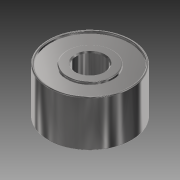
# Autodesk Inventor part: bearing_693
Saved by Autodesk Inventor 2013 (Build 170138000, 138)
## iProperties
Shininess: 86.0
Created: 2011-05-14
Part Number: bearing_693
Document SubType Name: Modeling
Designer: Noa Izumi
Material: Default
Density: 1 g/cm^3
Density: 0.0
Volumn: 0.0
Area: 0.0
PropertySet Name: Model Information
Control State: 0
Master: False
Checked Out: False
Author: Noa Izumi
Autodesk Inventor part; units mm, degrees
ref_plane "YZ Plane" through (0, 0, 0) normal (1, 0, 0) x (0, 1, 0)
ref_plane "XZ Plane" through (0, 0, 0) normal (0, 1, 0) x (-1, 0, 0)
ref_plane "XY Plane" through (0, 0, 0) normal (0, 0, 1) x (1, 0, 0)
sketch "Sketch1" plane through (0, 0, 0) normal (0, 0, 1) x (1, 0, 0)
  circle A0 centre (0, 0) radius 4.5
  circle A1 centre (0, 0) radius 1.5
  dimension "d0" = 9
  dimension "d1" = 3
  constraints: 2 centre point, 1 coincident
  measures "d0" diameter of A0
  measures "d1" diameter of A1
extrude "Extrusion1" add sketch "Sketch1" along normal blind 5
sketch "Sketch2" plane through (0, 0, 5) normal (0, 0, 1) x (1, 0, 0)
  circle A0 centre (0, 0) radius 4.5 projected
  circle A1 centre (0, 0) radius 2.5
  circle A2 centre (0, 0) radius 4.25
  dimension "d4" = 8.5
  dimension "d5" = 5
  constraints: 2 centre point, 2 coincident
  measures "d4" diameter of A2
  measures "d5" diameter of A1
extrude "Extrusion2" cut sketch "Sketch2" against normal blind 0.25 contours A2
sketch "Sketch3" plane through (0, 0, 0) normal (0, 0, -1) x (-1, 0, 0)
  circle A0 centre (0, 0) radius 4.5 projected
  circle A1 centre (0, 0) radius 2.5
  circle A2 centre (0, 0) radius 4.25
  dimension "d8" = 5
  dimension "d9" = 8.5
  constraints: 2 centre point, 2 coincident
  measures "d8" diameter of A1
  measures "d9" diameter of A2
extrude "Extrusion3" cut sketch "Sketch3" against normal blind 0.25 contours A2
fillet "Fillet1" radius 0.125 6 edges at (-4.5, 0, 0) (4.25, 0, 0) (-4.5, 0, 5) (-4.25, 0, 5) (2.5, 0, 0) (-2.5, 0, 5)
chamfer "Chamfer1" distance 0.125 angle 45 2 edges at (-1.5, 0, 5) (-1.5, 0, 0)
